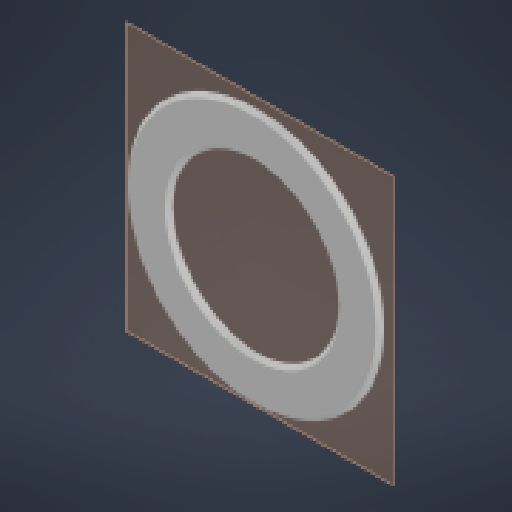
# Autodesk Inventor part: OuterRing
Saved by Autodesk Inventor 2023 (Build 270158000, 158)
## iProperties
Created: 2023-08-14
Part Number: OuterRing
Material: Generic
Document SubType Name: Modeling
Designer: Izack Waczko
Density: 1 g/cm^3
Appearance: Default
Author: Izack Waczko
Autodesk Inventor part; units mm, degrees
ref_plane "YZ Plane" through (0, 0, 0) normal (1, 0, 0) x (0, 1, 0)
ref_plane "XZ Plane" through (0, 0, 0) normal (0, 1, 0) x (-1, 0, 0)
ref_plane "XY Plane" through (0, 0, 0) normal (0, 0, 1) x (1, 0, 0)
ref_plane "Work Plane1" through (0, 0, 0) normal (0, 0, 1) x (1, 0, 0)
sketch "Sketch1" plane through (0, 0, 0) normal (0, 0, 1) x (1, 0, 0)
  arc A0 (-18.4196, 18.1475) -> (-12.6086, 22.5751) centre (-15, 19.6866) ccw
  arc A1 (6.8192, 37.3831) -> (6.0242, 37.5195) centre (0, 0) ccw
  arc A2 (6.0242, 37.5195) -> (4.917, 35.4102) centre (17.1774, 30.3196) ccw
  arc A3 (4.917, 35.4102) -> (4.1643, 35.5066) centre (0, 0) ccw
  arc A4 (4.1643, 35.5066) -> (3.6243, 37.8268) centre (-8.9833, 33.6696) ccw
  arc A5 (3.6243, 37.8268) -> (2.8206, 37.8952) centre (0, 0) ccw
  arc A6 (2.8206, 37.8952) -> (1.8963, 35.6997) centre (14.5443, 31.6671) ccw
  arc A7 (1.8963, 35.6997) -> (1.1381, 35.7319) centre (0, 0) ccw
  arc A8 (1.1381, 35.7319) -> (0.4033, 37.9979) centre (-11.8063, 32.7865) ccw
  arc A9 (0.4033, 37.9979) -> (-0.4033, 37.9979) centre (0, 0) ccw
  arc A10 (-0.4033, 37.9979) -> (-1.1381, 35.7319) centre (11.8063, 32.7865) ccw
  arc A11 (-1.1381, 35.7319) -> (-1.8963, 35.6997) centre (0, 0) ccw
  arc A12 (-1.8963, 35.6997) -> (-2.8206, 37.8952) centre (-14.5443, 31.6671) ccw
  arc A13 (-2.8206, 37.8952) -> (-3.6243, 37.8268) centre (0, 0) ccw
  arc A14 (-3.6243, 37.8268) -> (-4.1643, 35.5066) centre (8.9833, 33.6696) ccw
  arc A15 (-4.1643, 35.5066) -> (-4.917, 35.4102) centre (0, 0) ccw
  arc A16 (-4.917, 35.4102) -> (-6.0242, 37.5195) centre (-17.1774, 30.3196) ccw
  arc A17 (-6.0242, 37.5195) -> (-6.8192, 37.3831) centre (0, 0) ccw
  arc A18 (-6.8192, 37.3831) -> (-7.1605, 35.0256) centre (6.0955, 34.3101) ccw
  arc A19 (-7.1605, 35.0256) -> (-7.9023, 34.8657) centre (0, 0) ccw
  arc A20 (-7.9023, 34.8657) -> (-9.1843, 36.8734) centre (-19.6868, 28.7536) ccw
  arc A21 (-9.1843, 36.8734) -> (-9.9649, 36.6702) centre (0, 0) ccw
  arc A22 (-9.9649, 36.6702) -> (-10.105, 34.2921) centre (3.1639, 34.7035) ccw
  arc A23 (-10.105, 34.2921) -> (-10.8306, 34.0699) centre (0, 0) ccw
  arc A24 (-10.8306, 34.0699) -> (-12.2783, 35.9617) centre (-22.0544, 26.9805) ccw
  arc A25 (-12.2783, 35.9617) -> (-13.0389, 35.693) centre (0, 0) ccw
  arc A26 (-13.0389, 35.693) -> (-12.9768, 33.3116) centre (0.2094, 34.8468) ccw
  arc A27 (-12.9768, 33.3116) -> (-13.6809, 33.0287) centre (0, 0) ccw
  arc A28 (-13.6809, 33.0287) -> (-15.2839, 34.7909) centre (-24.263, 25.0129) ccw
  arc A29 (-15.2839, 34.7909) -> (-16.0189, 34.4586) centre (0, 0) ccw
  arc A30 (-16.0189, 34.4586) -> (-15.7551, 32.0911) centre (-2.7465, 34.739) ccw
  arc A31 (-15.7551, 32.0911) -> (-16.4327, 31.7495) centre (0, 0) ccw
  arc A32 (-16.4327, 31.7495) -> (-18.1793, 33.3694) centre (-26.2969, 22.8652) ccw
  arc A33 (-18.1793, 33.3694) -> (-18.8835, 32.976) centre (0, 0) ccw
  arc A34 (-18.8835, 32.976) -> (-18.4198, 30.6394) centre (-5.6827, 34.3809) ccw
  arc A35 (-18.4198, 30.6394) -> (-19.066, 30.2415) centre (0, 0) ccw
  arc A36 (-19.066, 30.2415) -> (-20.9437, 31.7074) centre (-28.1412, 20.5527) ccw
  arc A37 (-20.9437, 31.7074) -> (-21.612, 31.2558) centre (0, 0) ccw
  arc A38 (-21.612, 31.2558) -> (-20.9519, 28.9669) centre (-8.578, 33.7751) ccw
  arc A39 (-20.9519, 28.9669) -> (-21.562, 28.5157) centre (0, 0) ccw
  arc A40 (-21.562, 28.5157) -> (-23.5572, 29.8171) centre (-29.7828, 18.0921) ccw
  arc A41 (-23.5572, 29.8171) -> (-24.1848, 29.3103) centre (0, 0) ccw
  arc A42 (-24.1848, 29.3103) -> (-23.333, 27.0857) centre (-11.4114, 32.926) ccw
  arc A43 (-23.333, 27.0857) -> (-23.9026, 26.5843) centre (0, 0) ccw
  arc A44 (-23.9026, 26.5843) -> (-26.001, 27.7118) centre (-31.2099, 15.5011) ccw
  arc A45 (-26.001, 27.7118) -> (-26.5834, 27.1537) centre (0, 0) ccw
  arc A46 (-26.5834, 27.1537) -> (-25.5459, 25.0093) centre (-14.1626, 31.8396) ccw
  arc A47 (-25.5459, 25.0093) -> (-26.071, 24.4615) centre (0, 0) ccw
  arc A48 (-26.071, 24.4615) -> (-28.2575, 25.407) centre (-32.412, 12.7985) ccw
  arc A49 (-28.2575, 25.407) -> (-28.7904, 24.8015) centre (0, 0) ccw
  arc A50 (-28.7904, 24.8015) -> (-27.5748, 22.7528) centre (-16.8118, 30.5239) ccw
  arc A51 (-27.5748, 22.7528) -> (-28.0516, 22.1624) centre (0, 0) ccw
  arc A52 (-28.0516, 22.1624) -> (-30.3104, 22.919) centre (-33.3806, 10.0037) ccw
  arc A53 (-30.3104, 22.919) -> (-30.79, 22.2705) centre (0, 0) ccw
  arc A54 (-30.79, 22.2705) -> (-29.4051, 20.3323) centre (-19.3398, 28.9882) ccw
  arc A55 (-29.4051, 20.3323) -> (-29.83, 19.7036) centre (0, 0) ccw
  arc A56 (-29.83, 19.7036) -> (-32.1448, 20.266) centre (-34.1088, 7.1368) ccw
  arc A57 (-32.1448, 20.266) -> (-32.5677, 19.5791) centre (0, 0) ccw
  arc A58 (-32.5677, 19.5791) -> (-31.0235, 17.7654) centre (-21.7285, 27.2436) ccw
  arc A59 (-31.0235, 17.7654) -> (-31.3935, 17.1029) centre (0, 0) ccw
  arc A60 (-31.3935, 17.1029) -> (-33.7477, 17.4669) centre (-34.5911, 4.2184) ccw
  arc A61 (-33.7477, 17.4669) -> (-34.1108, 16.7467) centre (0, 0) ccw
  arc A62 (-34.1108, 16.7467) -> (-32.4183, 15.0704) centre (-23.9606, 25.3027) ccw
  arc A63 (-32.4183, 15.0704) -> (-32.7309, 14.3789) centre (0, 0) ccw
  arc A64 (-32.7309, 14.3789) -> (-35.1074, 14.542) centre (-34.8243, 1.2697) ccw
  arc A65 (-35.1074, 14.542) -> (-35.4082, 13.7935) centre (0, 0) ccw
  arc A66 (-35.4082, 13.7935) -> (-33.5796, 12.2668) centre (-26.0201, 23.1796) ccw
  arc A67 (-33.5796, 12.2668) -> (-33.8324, 11.5513) centre (0, 0) ccw
  arc A68 (-33.8324, 11.5513) -> (-36.2142, 11.5123) centre (-34.8065, -1.6882) ccw
  arc A69 (-36.2142, 11.5123) -> (-36.4504, 10.741) centre (0, 0) ccw
  arc A70 (-36.4504, 10.741) -> (-34.4989, 9.3749) centre (-27.8922, 20.8894) ccw
  arc A71 (-34.4989, 9.3749) -> (-34.6901, 8.6405) centre (0, 0) ccw
  arc A72 (-34.6901, 8.6405) -> (-37.06, 8.3996) centre (-34.5379, -4.6339) ccw
  arc A73 (-37.06, 8.3996) -> (-37.23, 7.6111) centre (0, 0) ccw
  arc A74 (-37.23, 7.6111) -> (-35.1697, 6.4154) centre (-29.5632, 18.4487) ccw
  arc A75 (-35.1697, 6.4154) -> (-35.2979, 5.6675) centre (0, 0) ccw
  arc A76 (-35.2979, 5.6675) -> (-37.6389, 5.2264) centre (-34.0205, -7.5462) ccw
  arc A77 (-37.6389, 5.2264) -> (-37.7413, 4.4264) centre (0, 0) ccw
  arc A78 (-37.7413, 4.4264) -> (-35.587, 3.4097) centre (-31.0213, 15.8751) ccw
  arc A79 (-35.587, 3.4097) -> (-35.6514, 2.6536) centre (0, 0) ccw
  arc A80 (-35.6514, 2.6536) -> (-37.9465, 2.0156) centre (-33.258, -10.4042) ccw
  arc A81 (-37.9465, 2.0156) -> (-37.9807, 1.2097) centre (0, 0) ccw
  arc A82 (-37.9807, 1.2097) -> (-35.748, 0.3794) centre (-32.2559, 13.1872) ccw
  arc A83 (-35.748, 0.3794) -> (-35.748, -0.3794) centre (0, 0) ccw
  arc A84 (-35.748, -0.3794) -> (-37.9807, -1.2097) centre (-32.2559, -13.1872) ccw
  arc A85 (-37.9807, -1.2097) -> (-37.9465, -2.0156) centre (0, 0) ccw
  arc A86 (-37.9465, -2.0156) -> (-35.6514, -2.6536) centre (-33.258, 10.4042) ccw
  arc A87 (-35.6514, -2.6536) -> (-35.587, -3.4097) centre (0, 0) ccw
  arc A88 (-35.587, -3.4097) -> (-37.7413, -4.4264) centre (-31.0213, -15.8751) ccw
  arc A89 (-37.7413, -4.4264) -> (-37.6389, -5.2264) centre (0, 0) ccw
  arc A90 (-37.6389, -5.2264) -> (-35.2979, -5.6675) centre (-34.0205, 7.5462) ccw
  arc A91 (-35.2979, -5.6675) -> (-35.1697, -6.4154) centre (0, 0) ccw
  arc A92 (-35.1697, -6.4154) -> (-37.23, -7.6111) centre (-29.5632, -18.4487) ccw
  arc A93 (-37.23, -7.6111) -> (-37.06, -8.3996) centre (0, 0) ccw
  arc A94 (-37.06, -8.3996) -> (-34.6901, -8.6405) centre (-34.5379, 4.6339) ccw
  arc A95 (-34.6901, -8.6405) -> (-34.4989, -9.3749) centre (0, 0) ccw
  arc A96 (-34.4989, -9.3749) -> (-36.4504, -10.741) centre (-27.8922, -20.8894) ccw
  arc A97 (-36.4504, -10.741) -> (-36.2142, -11.5123) centre (0, 0) ccw
  arc A98 (-36.2142, -11.5123) -> (-33.8324, -11.5513) centre (-34.8065, 1.6882) ccw
  arc A99 (-33.8324, -11.5513) -> (-33.5796, -12.2668) centre (0, 0) ccw
  arc A100 (-33.5796, -12.2668) -> (-35.4082, -13.7935) centre (-26.0201, -23.1796) ccw
  arc A101 (-35.4082, -13.7935) -> (-35.1074, -14.542) centre (0, 0) ccw
  arc A102 (-35.1074, -14.542) -> (-32.7309, -14.3789) centre (-34.8243, -1.2697) ccw
  arc A103 (-32.7309, -14.3789) -> (-32.4183, -15.0704) centre (0, 0) ccw
  arc A104 (-32.4183, -15.0704) -> (-34.1108, -16.7467) centre (-23.9606, -25.3027) ccw
  arc A105 (-34.1108, -16.7467) -> (-33.7477, -17.4669) centre (0, 0) ccw
  arc A106 (-33.7477, -17.4669) -> (-31.3935, -17.1029) centre (-34.5911, -4.2184) ccw
  arc A107 (-31.3935, -17.1029) -> (-31.0235, -17.7654) centre (0, 0) ccw
  arc A108 (-31.0235, -17.7654) -> (-32.5677, -19.5791) centre (-21.7285, -27.2436) ccw
  arc A109 (-32.5677, -19.5791) -> (-32.1448, -20.266) centre (0, 0) ccw
  arc A110 (-32.1448, -20.266) -> (-29.83, -19.7036) centre (-34.1088, -7.1368) ccw
  arc A111 (-29.83, -19.7036) -> (-29.4051, -20.3323) centre (0, 0) ccw
  arc A112 (-29.4051, -20.3323) -> (-30.79, -22.2705) centre (-19.3398, -28.9882) ccw
  arc A113 (-30.79, -22.2705) -> (-30.3104, -22.919) centre (0, 0) ccw
  arc A114 (-30.3104, -22.919) -> (-28.0516, -22.1624) centre (-33.3806, -10.0037) ccw
  arc A115 (-28.0516, -22.1624) -> (-27.5748, -22.7528) centre (0, 0) ccw
  arc A116 (-27.5748, -22.7528) -> (-28.7904, -24.8015) centre (-16.8118, -30.5239) ccw
  arc A117 (-28.7904, -24.8015) -> (-28.2575, -25.407) centre (0, 0) ccw
  arc A118 (-28.2575, -25.407) -> (-26.071, -24.4615) centre (-32.412, -12.7985) ccw
  arc A119 (-26.071, -24.4615) -> (-25.5459, -25.0093) centre (0, 0) ccw
  arc A120 (-25.5459, -25.0093) -> (-26.5834, -27.1537) centre (-14.1626, -31.8396) ccw
  arc A121 (-26.5834, -27.1537) -> (-26.001, -27.7118) centre (0, 0) ccw
  arc A122 (-26.001, -27.7118) -> (-23.9026, -26.5843) centre (-31.2099, -15.5011) ccw
  arc A123 (-23.9026, -26.5843) -> (-23.333, -27.0857) centre (0, 0) ccw
  arc A124 (-23.333, -27.0857) -> (-24.1848, -29.3103) centre (-11.4114, -32.926) ccw
  arc A125 (-24.1848, -29.3103) -> (-23.5572, -29.8171) centre (0, 0) ccw
  arc A126 (-23.5572, -29.8171) -> (-21.562, -28.5157) centre (-29.7828, -18.0921) ccw
  arc A127 (-21.562, -28.5157) -> (-20.9519, -28.9669) centre (0, 0) ccw
  arc A128 (-20.9519, -28.9669) -> (-21.612, -31.2558) centre (-8.578, -33.7751) ccw
  arc A129 (-21.612, -31.2558) -> (-20.9437, -31.7074) centre (0, 0) ccw
  arc A130 (-20.9437, -31.7074) -> (-19.066, -30.2415) centre (-28.1412, -20.5527) ccw
  arc A131 (-19.066, -30.2415) -> (-18.4198, -30.6394) centre (0, 0) ccw
  arc A132 (-18.4198, -30.6394) -> (-18.8835, -32.976) centre (-5.6827, -34.3809) ccw
  arc A133 (-18.8835, -32.976) -> (-18.1793, -33.3694) centre (0, 0) ccw
  arc A134 (-18.1793, -33.3694) -> (-16.4327, -31.7495) centre (-26.2969, -22.8652) ccw
  arc A135 (-16.4327, -31.7495) -> (-15.7551, -32.0911) centre (0, 0) ccw
  arc A136 (-15.7551, -32.0911) -> (-16.0189, -34.4586) centre (-2.7465, -34.739) ccw
  arc A137 (-16.0189, -34.4586) -> (-15.2839, -34.7909) centre (0, 0) ccw
  arc A138 (-15.2839, -34.7909) -> (-13.6809, -33.0287) centre (-24.263, -25.0129) ccw
  arc A139 (-13.6809, -33.0287) -> (-12.9768, -33.3116) centre (0, 0) ccw
  arc A140 (-12.9768, -33.3116) -> (-13.0389, -35.693) centre (0.2094, -34.8468) ccw
  arc A141 (-13.0389, -35.693) -> (-12.2783, -35.9617) centre (0, 0) ccw
  arc A142 (-12.2783, -35.9617) -> (-10.8306, -34.0699) centre (-22.0544, -26.9805) ccw
  arc A143 (-10.8306, -34.0699) -> (-10.105, -34.2921) centre (0, 0) ccw
  arc A144 (-10.105, -34.2921) -> (-9.9649, -36.6702) centre (3.1639, -34.7035) ccw
  arc A145 (-9.9649, -36.6702) -> (-9.1843, -36.8734) centre (0, 0) ccw
  arc A146 (-9.1843, -36.8734) -> (-7.9023, -34.8657) centre (-19.6868, -28.7536) ccw
  arc A147 (-7.9023, -34.8657) -> (-7.1605, -35.0256) centre (0, 0) ccw
  arc A148 (-7.1605, -35.0256) -> (-6.8192, -37.3831) centre (6.0955, -34.3101) ccw
  arc A149 (-6.8192, -37.3831) -> (-6.0242, -37.5195) centre (0, 0) ccw
  arc A150 (-6.0242, -37.5195) -> (-4.917, -35.4102) centre (-17.1774, -30.3196) ccw
  arc A151 (-4.917, -35.4102) -> (-4.1643, -35.5066) centre (0, 0) ccw
  arc A152 (-4.1643, -35.5066) -> (-3.6243, -37.8268) centre (8.9833, -33.6696) ccw
  arc A153 (-3.6243, -37.8268) -> (-2.8206, -37.8952) centre (0, 0) ccw
  arc A154 (-2.8206, -37.8952) -> (-1.8963, -35.6997) centre (-14.5443, -31.6671) ccw
  arc A155 (-1.8963, -35.6997) -> (-1.1381, -35.7319) centre (0, 0) ccw
  arc A156 (-1.1381, -35.7319) -> (-0.4033, -37.9979) centre (11.8063, -32.7865) ccw
  arc A157 (-0.4033, -37.9979) -> (0.4033, -37.9979) centre (0, 0) ccw
  arc A158 (0.4033, -37.9979) -> (1.1381, -35.7319) centre (-11.8063, -32.7865) ccw
  arc A159 (1.1381, -35.7319) -> (1.8963, -35.6997) centre (0, 0) ccw
  arc A160 (1.8963, -35.6997) -> (2.8206, -37.8952) centre (14.5443, -31.6671) ccw
  arc A161 (2.8206, -37.8952) -> (3.6243, -37.8268) centre (0, 0) ccw
  arc A162 (3.6243, -37.8268) -> (4.1643, -35.5066) centre (-8.9833, -33.6696) ccw
  arc A163 (4.1643, -35.5066) -> (4.917, -35.4102) centre (0, 0) ccw
  arc A164 (4.917, -35.4102) -> (6.0242, -37.5195) centre (17.1774, -30.3196) ccw
  arc A165 (6.0242, -37.5195) -> (6.8192, -37.3831) centre (0, 0) ccw
  arc A166 (6.8192, -37.3831) -> (7.1605, -35.0256) centre (-6.0955, -34.3101) ccw
  arc A167 (7.1605, -35.0256) -> (7.9023, -34.8657) centre (0, 0) ccw
  arc A168 (7.9023, -34.8657) -> (9.1843, -36.8734) centre (19.6868, -28.7536) ccw
  arc A169 (9.1843, -36.8734) -> (9.9649, -36.6702) centre (0, 0) ccw
  arc A170 (9.9649, -36.6702) -> (10.105, -34.2921) centre (-3.1639, -34.7035) ccw
  arc A171 (10.105, -34.2921) -> (10.8306, -34.0699) centre (0, 0) ccw
  arc A172 (10.8306, -34.0699) -> (12.2783, -35.9617) centre (22.0544, -26.9805) ccw
  arc A173 (12.2783, -35.9617) -> (13.0389, -35.693) centre (0, 0) ccw
  arc A174 (13.0389, -35.693) -> (12.9768, -33.3116) centre (-0.2094, -34.8468) ccw
  arc A175 (12.9768, -33.3116) -> (13.6809, -33.0287) centre (0, 0) ccw
  arc A176 (13.6809, -33.0287) -> (15.2839, -34.7909) centre (24.263, -25.0129) ccw
  arc A177 (15.2839, -34.7909) -> (16.0189, -34.4586) centre (0, 0) ccw
  arc A178 (16.0189, -34.4586) -> (15.7551, -32.0911) centre (2.7465, -34.739) ccw
  arc A179 (15.7551, -32.0911) -> (16.4327, -31.7495) centre (0, 0) ccw
  arc A180 (16.4327, -31.7495) -> (18.1793, -33.3694) centre (26.2969, -22.8652) ccw
  arc A181 (18.1793, -33.3694) -> (18.8835, -32.976) centre (0, 0) ccw
  arc A182 (18.8835, -32.976) -> (18.4198, -30.6394) centre (5.6827, -34.3809) ccw
  arc A183 (18.4198, -30.6394) -> (19.066, -30.2415) centre (0, 0) ccw
  arc A184 (19.066, -30.2415) -> (20.9437, -31.7074) centre (28.1412, -20.5527) ccw
  arc A185 (20.9437, -31.7074) -> (21.612, -31.2558) centre (0, 0) ccw
  arc A186 (21.612, -31.2558) -> (20.9519, -28.9669) centre (8.578, -33.7751) ccw
  arc A187 (20.9519, -28.9669) -> (21.562, -28.5157) centre (0, 0) ccw
  arc A188 (21.562, -28.5157) -> (23.5572, -29.8171) centre (29.7828, -18.0921) ccw
  arc A189 (23.5572, -29.8171) -> (24.1848, -29.3103) centre (0, 0) ccw
  arc A190 (24.1848, -29.3103) -> (23.333, -27.0857) centre (11.4114, -32.926) ccw
  arc A191 (23.333, -27.0857) -> (23.9026, -26.5843) centre (0, 0) ccw
  arc A192 (23.9026, -26.5843) -> (26.001, -27.7118) centre (31.2099, -15.5011) ccw
  arc A193 (26.001, -27.7118) -> (26.5834, -27.1537) centre (0, 0) ccw
  arc A194 (26.5834, -27.1537) -> (25.5459, -25.0093) centre (14.1626, -31.8396) ccw
  arc A195 (25.5459, -25.0093) -> (26.071, -24.4615) centre (0, 0) ccw
  arc A196 (26.071, -24.4615) -> (28.2575, -25.407) centre (32.412, -12.7985) ccw
  arc A197 (28.2575, -25.407) -> (28.7904, -24.8015) centre (0, 0) ccw
  arc A198 (28.7904, -24.8015) -> (27.5748, -22.7528) centre (16.8118, -30.5239) ccw
  arc A199 (27.5748, -22.7528) -> (28.0516, -22.1624) centre (0, 0) ccw
  arc A200 (28.0516, -22.1624) -> (30.3104, -22.919) centre (33.3806, -10.0037) ccw
  arc A201 (30.3104, -22.919) -> (30.79, -22.2705) centre (0, 0) ccw
  arc A202 (30.79, -22.2705) -> (29.4051, -20.3323) centre (19.3398, -28.9882) ccw
  arc A203 (29.4051, -20.3323) -> (29.83, -19.7036) centre (0, 0) ccw
  arc A204 (29.83, -19.7036) -> (32.1448, -20.266) centre (34.1088, -7.1368) ccw
  arc A205 (32.1448, -20.266) -> (32.5677, -19.5791) centre (0, 0) ccw
  arc A206 (32.5677, -19.5791) -> (31.0235, -17.7654) centre (21.7285, -27.2436) ccw
  arc A207 (31.0235, -17.7654) -> (31.3935, -17.1029) centre (0, 0) ccw
  arc A208 (31.3935, -17.1029) -> (33.7477, -17.4669) centre (34.5911, -4.2184) ccw
  arc A209 (33.7477, -17.4669) -> (34.1108, -16.7467) centre (0, 0) ccw
  arc A210 (34.1108, -16.7467) -> (32.4183, -15.0704) centre (23.9606, -25.3027) ccw
  arc A211 (32.4183, -15.0704) -> (32.7309, -14.3789) centre (0, 0) ccw
  arc A212 (32.7309, -14.3789) -> (35.1074, -14.542) centre (34.8243, -1.2697) ccw
  arc A213 (35.1074, -14.542) -> (35.4082, -13.7935) centre (0, 0) ccw
  arc A214 (35.4082, -13.7935) -> (33.5796, -12.2668) centre (26.0201, -23.1796) ccw
  arc A215 (33.5796, -12.2668) -> (33.8324, -11.5513) centre (0, 0) ccw
  arc A216 (33.8324, -11.5513) -> (36.2142, -11.5123) centre (34.8065, 1.6882) ccw
  arc A217 (36.2142, -11.5123) -> (36.4504, -10.741) centre (0, 0) ccw
  arc A218 (36.4504, -10.741) -> (34.4989, -9.3749) centre (27.8922, -20.8894) ccw
  arc A219 (34.4989, -9.3749) -> (34.6901, -8.6405) centre (0, 0) ccw
  arc A220 (34.6901, -8.6405) -> (37.06, -8.3996) centre (34.5379, 4.6339) ccw
  arc A221 (37.06, -8.3996) -> (37.23, -7.6111) centre (0, 0) ccw
  arc A222 (37.23, -7.6111) -> (35.1697, -6.4154) centre (29.5632, -18.4487) ccw
  arc A223 (35.1697, -6.4154) -> (35.2979, -5.6675) centre (0, 0) ccw
  arc A224 (35.2979, -5.6675) -> (37.6389, -5.2264) centre (34.0205, 7.5462) ccw
  arc A225 (37.6389, -5.2264) -> (37.7413, -4.4264) centre (0, 0) ccw
  arc A226 (37.7413, -4.4264) -> (35.587, -3.4097) centre (31.0213, -15.8751) ccw
  arc A227 (35.587, -3.4097) -> (35.6514, -2.6536) centre (0, 0) ccw
  arc A228 (35.6514, -2.6536) -> (37.9465, -2.0156) centre (33.258, 10.4042) ccw
  arc A229 (37.9465, -2.0156) -> (37.9807, -1.2097) centre (0, 0) ccw
  arc A230 (37.9807, -1.2097) -> (35.748, -0.3794) centre (32.2559, -13.1872) ccw
  arc A231 (35.748, -0.3794) -> (35.748, 0.3794) centre (0, 0) ccw
  arc A232 (35.748, 0.3794) -> (37.9807, 1.2097) centre (32.2559, 13.1872) ccw
  arc A233 (37.9807, 1.2097) -> (37.9465, 2.0156) centre (0, 0) ccw
  arc A234 (37.9465, 2.0156) -> (35.6514, 2.6536) centre (33.258, -10.4042) ccw
  arc A235 (35.6514, 2.6536) -> (35.587, 3.4097) centre (0, 0) ccw
  arc A236 (35.587, 3.4097) -> (37.7413, 4.4264) centre (31.0213, 15.8751) ccw
  arc A237 (37.7413, 4.4264) -> (37.6389, 5.2264) centre (0, 0) ccw
  arc A238 (37.6389, 5.2264) -> (35.2979, 5.6675) centre (34.0205, -7.5462) ccw
  arc A239 (35.2979, 5.6675) -> (35.1697, 6.4154) centre (0, 0) ccw
  arc A240 (35.1697, 6.4154) -> (37.23, 7.6111) centre (29.5632, 18.4487) ccw
  arc A241 (37.23, 7.6111) -> (37.06, 8.3996) centre (0, 0) ccw
  arc A242 (37.06, 8.3996) -> (34.6901, 8.6405) centre (34.5379, -4.6339) ccw
  arc A243 (34.6901, 8.6405) -> (34.4989, 9.3749) centre (0, 0) ccw
  arc A244 (34.4989, 9.3749) -> (36.4504, 10.741) centre (27.8922, 20.8894) ccw
  arc A245 (36.4504, 10.741) -> (36.2142, 11.5123) centre (0, 0) ccw
  arc A246 (36.2142, 11.5123) -> (33.8324, 11.5513) centre (34.8065, -1.6882) ccw
  arc A247 (33.8324, 11.5513) -> (33.5796, 12.2668) centre (0, 0) ccw
  arc A248 (33.5796, 12.2668) -> (35.4082, 13.7935) centre (26.0201, 23.1796) ccw
  arc A249 (35.4082, 13.7935) -> (35.1074, 14.542) centre (0, 0) ccw
  arc A250 (35.1074, 14.542) -> (32.7309, 14.3789) centre (34.8243, 1.2697) ccw
  arc A251 (32.7309, 14.3789) -> (32.4183, 15.0704) centre (0, 0) ccw
  arc A252 (32.4183, 15.0704) -> (34.1108, 16.7467) centre (23.9606, 25.3027) ccw
  arc A253 (34.1108, 16.7467) -> (33.7477, 17.4669) centre (0, 0) ccw
  arc A254 (33.7477, 17.4669) -> (31.3935, 17.1029) centre (34.5911, 4.2184) ccw
  arc A255 (31.3935, 17.1029) -> (31.0235, 17.7654) centre (0, 0) ccw
  arc A256 (31.0235, 17.7654) -> (32.5677, 19.5791) centre (21.7285, 27.2436) ccw
  arc A257 (32.5677, 19.5791) -> (32.1448, 20.266) centre (0, 0) ccw
  arc A258 (32.1448, 20.266) -> (29.83, 19.7036) centre (34.1088, 7.1368) ccw
  arc A259 (29.83, 19.7036) -> (29.4051, 20.3323) centre (0, 0) ccw
  arc A260 (29.4051, 20.3323) -> (30.79, 22.2705) centre (19.3398, 28.9882) ccw
  arc A261 (30.79, 22.2705) -> (30.3104, 22.919) centre (0, 0) ccw
  arc A262 (30.3104, 22.919) -> (28.0516, 22.1624) centre (33.3806, 10.0037) ccw
  arc A263 (28.0516, 22.1624) -> (27.5748, 22.7528) centre (0, 0) ccw
  arc A264 (27.5748, 22.7528) -> (28.7904, 24.8015) centre (16.8118, 30.5239) ccw
  arc A265 (28.7904, 24.8015) -> (28.2575, 25.407) centre (0, 0) ccw
  arc A266 (28.2575, 25.407) -> (26.071, 24.4615) centre (32.412, 12.7985) ccw
  arc A267 (26.071, 24.4615) -> (25.5459, 25.0093) centre (0, 0) ccw
  arc A268 (25.5459, 25.0093) -> (26.5834, 27.1537) centre (14.1626, 31.8396) ccw
  arc A269 (26.5834, 27.1537) -> (26.001, 27.7118) centre (0, 0) ccw
  arc A270 (26.001, 27.7118) -> (23.9026, 26.5843) centre (31.2099, 15.5011) ccw
  arc A271 (23.9026, 26.5843) -> (23.333, 27.0857) centre (0, 0) ccw
  arc A272 (23.333, 27.0857) -> (24.1848, 29.3103) centre (11.4114, 32.926) ccw
  arc A273 (24.1848, 29.3103) -> (23.5572, 29.8171) centre (0, 0) ccw
  arc A274 (23.5572, 29.8171) -> (21.562, 28.5157) centre (29.7828, 18.0921) ccw
  arc A275 (21.562, 28.5157) -> (20.9519, 28.9669) centre (0, 0) ccw
  arc A276 (20.9519, 28.9669) -> (21.612, 31.2558) centre (8.578, 33.7751) ccw
  arc A277 (21.612, 31.2558) -> (20.9437, 31.7074) centre (0, 0) ccw
  arc A278 (20.9437, 31.7074) -> (19.066, 30.2415) centre (28.1412, 20.5527) ccw
  arc A279 (19.066, 30.2415) -> (18.4198, 30.6394) centre (0, 0) ccw
  arc A280 (18.4198, 30.6394) -> (18.8835, 32.976) centre (5.6827, 34.3809) ccw
  arc A281 (18.8835, 32.976) -> (18.1793, 33.3694) centre (0, 0) ccw
  arc A282 (18.1793, 33.3694) -> (16.4327, 31.7495) centre (26.2969, 22.8652) ccw
  arc A283 (16.4327, 31.7495) -> (15.7551, 32.0911) centre (0, 0) ccw
  arc A284 (15.7551, 32.0911) -> (16.0189, 34.4586) centre (2.7465, 34.739) ccw
  arc A285 (16.0189, 34.4586) -> (15.2839, 34.7909) centre (0, 0) ccw
  arc A286 (15.2839, 34.7909) -> (13.6809, 33.0287) centre (24.263, 25.0129) ccw
  arc A287 (13.6809, 33.0287) -> (12.9768, 33.3116) centre (0, 0) ccw
  arc A288 (12.9768, 33.3116) -> (13.0389, 35.693) centre (-0.2094, 34.8468) ccw
  arc A289 (13.0389, 35.693) -> (12.2783, 35.9617) centre (0, 0) ccw
  arc A290 (12.2783, 35.9617) -> (10.8306, 34.0699) centre (22.0544, 26.9805) ccw
  arc A291 (10.8306, 34.0699) -> (10.105, 34.2921) centre (0, 0) ccw
  arc A292 (10.105, 34.2921) -> (9.9649, 36.6702) centre (-3.1639, 34.7035) ccw
  arc A293 (9.9649, 36.6702) -> (9.1843, 36.8734) centre (0, 0) ccw
  arc A294 (9.1843, 36.8734) -> (7.9023, 34.8657) centre (19.6868, 28.7536) ccw
  arc A295 (7.9023, 34.8657) -> (7.1605, 35.0256) centre (0, 0) ccw
  arc A296 (7.1605, 35.0256) -> (6.8192, 37.3831) centre (-6.0955, 34.3101) ccw
  arc A297 (26.0035, 11.6649) -> (18.1475, 21.9754) centre (0, 0) ccw
  arc A298 (26.0035, 11.6649) -> (18.1475, 21.9754) centre (0, 0) ccw
  arc A299 (-11.6649, 26.0035) -> (-21.9754, 18.1475) centre (0, 0) ccw
  arc A300 (-26.3963, -10.7464) -> (-17.3662, -22.5979) centre (0, 0) ccw
  arc A301 (11.6649, -26.0035) -> (21.9754, -18.1475) centre (0, 0) ccw
  circle A302 centre (0, 0) radius 40
  circle A303 centre (0, 0) radius 28.5
  circle A304 centre (0, 0) radius 25
  point P0 (0, 0)
extrude "Extrusion1" add sketch "Sketch1" along normal blind 1.25 contours A296 A295 A294 A293 A292 A291 A290 A289 A288 A287 A286 A285 A284 A283 A282 A281 A280 A279 A278 A277 A276 A275 A274 A273 A272 A271 A270 A269 A268 A267 A266 A265 A264 A263 A262 A261 A260 A259 A258 A257 A256 A255 A254 A253 A252 A251 A250 A249 A248 A247 A246 A245 A244 A243 A242 A241 A240 A239 A238 A237 A236 A235 A234 A233 A232 A231 A230 A229 A228 A227 A226 A225 A224 A223 A222 A221 A220 A219 A218 A217 A216 A215 A214 A213 A212 A211 A210 A209 A208 A207 A206 A205 A204 A203 A202 A201 A200 A199 A198 A197 A196 A195 A194 A193 A192 A191 A190 A189 A188 A187 A186 A185 A184 A183 A182 A181 A180 A179 A178 A177 A176 A175 A174 A173 A172 A171 A170 A169 A168 A167 A166 A165 A164 A163 A162 A161 A160 A159 A158 A157 A156 A155 A154 A153 A152 A151 A150 A149 A148 A147 A146 A145 A144 A143 A142 A141 A140 A139 A138 A137 A136 A135 A134 A133 A132 A131 A130 A129 A128 A127 A126 A125 A124 A123 A122 A121 A120 A119 A118 A117 A116 A115 A114 A113 A112 A111 A110 A109 A108 A107 A106 A105 A104 A103 A102 A101 A100 A99 A98 A97 A96 A95 A94 A93 A92 A91 A90 A89 A88 A87 A86 A85 A84 A83 A82 A81 A80 A79 A78 A77 A76 A75 A74 A73 A72 A71 A70 A69 A68 A67 A66 A65 A64 A63 A62 A61 A60 A59 A58 A57 A56 A55 A54 A53 A52 A51 A50 A49 A48 A47 A46 A45 A44 A43 A42 A41 A40 A39 A38 A37 A36 A35 A34 A33 A32 A31 A30 A29 A28 A27 A26 A25 A24 A23 A22 A21 A20 A19 A18 A17 A16 A15 A14 A13 A12 A11 A10 A9 A8 A7 A6 A5 A4 A3 A2 A1 | A303 A301 A300 A299 A297 | A302
chamfer "Chamfer2" distance 1.25 angle 45 2 edges at (-40, 0, 0) (-25, 0, 0)
body "Solid1"
